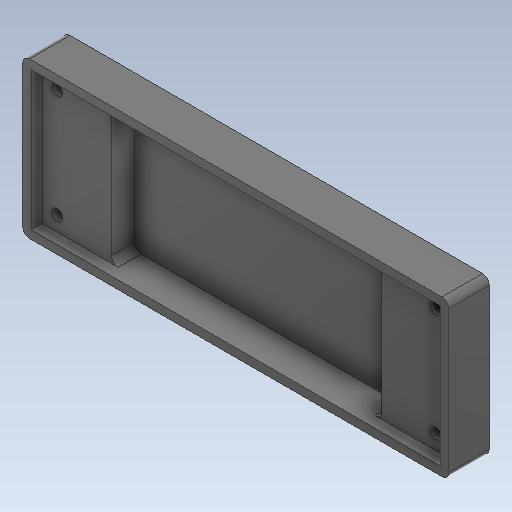
# Autodesk Inventor part: StartStopSwitch_cover_01
Saved by Autodesk Inventor 2020 (Build 240168000, 168)
## iProperties
Created: 2021-08-14
Part Number: StartStopSwitch_cover_01
Material: アセタール樹脂、黒
Document SubType Name: Modeling
Designer: Masato Kubotera
Density: 1.425 g/cm^3
Appearance: 滑らか - 黒
Mass: 5.48976 g
Surface Area: 46.7398 cm^2
Volume: 3.85246 cm^3
Author: Masato Kubotera
Title: StartStopSwitch_cover_01
Autodesk Inventor part; units mm, degrees
ref_plane "YZ Plane" through (0, 0, 0) normal (1, 0, 0) x (0, 1, 0)
ref_plane "XZ Plane" through (0, 0, 0) normal (0, 1, 0) x (-1, 0, 0)
ref_plane "XY Plane" through (0, 0, 0) normal (0, 0, 1) x (1, 0, 0)
sketch "スケッチ1" plane through (0, 0, 0) normal (0, 0, 1) x (1, 0, 0)
  line L0 (-31.5, 11.5) -> (31.5, 11.5)
  line L1 (31.5, 11.5) -> (31.5, -11.5)
  line L2 (31.5, -11.5) -> (-31.5, -11.5)
  line L3 (-31.5, -11.5) -> (-31.5, 11.5)
  line L4 (-31.5, 11.5) -> (31.5, -11.5) construction
  line L5 (31.5, 11.5) -> (-31.5, -11.5) construction
  line L6 (-30, 10) -> (30, 10) construction
  line L7 (30, 10) -> (30, -10) construction
  line L8 (30, -10) -> (-30, -10) construction
  line L9 (-30, -10) -> (-30, 10) construction
  line L10 (-30, 10) -> (30, -10) construction
  line L11 (30, 10) -> (-30, -10) construction
  circle A0 centre (-28, 8) radius 0.8
  line L12 (-31.5, 0) -> (31.5, 0) construction
  line L13 (0, 11.5) -> (0, -11.5) construction
  circle A1 centre (-28, -8) radius 0.8
  circle A2 centre (28, 8) radius 0.8
  circle A3 centre (28, -8) radius 0.8
  line L14 (-30.25, 10.25) -> (30.25, 10.25)
  line L15 (30.25, 10.25) -> (30.25, -10.25)
  line L16 (30.25, -10.25) -> (-30.25, -10.25)
  line L17 (-30.25, -10.25) -> (-30.25, 10.25)
  line L18 (-30.25, 10.25) -> (30.25, -10.25) construction
  line L19 (30.25, 10.25) -> (-30.25, -10.25) construction
  line L20 (-20, 10.25) -> (-20, -10.25)
  line L21 (20, 10.25) -> (20, -10.25)
  point P0 (0, 0)
  point P1 (0, 0)
  point P2 (20, -10.25)
  dimension "d0" = 63
  dimension "d1" = 60
  dimension "d2" = 20
  dimension "d3" = 23
  dimension "d4" = 1.6
  dimension "d5" = 2
  dimension "d6" = 2
  dimension "d7" = 20.5
  dimension "d8" = 60.5
  dimension "d13" = 10
  constraints: 44 end point, 12 midpoint, 6 parallel, 5 symmetric about line, 4 centre point, 4 perpendicular, 3 horizontal, 2 point on line, 3 other
  measures "d0" distance of L1.end L2.end
  measures "d1" distance of L7.end L8.end
  measures "d2" distance of L6.end L7.end
  measures "d3" distance of L0.end L1.end
  measures "d4" diameter of A0
  measures "d5" horizontal distance of A0.centre L6.start
  measures "d6" horizontal distance of A0.centre L6.start
  measures "d7" distance of L14.end L15.end
  measures "d8" distance of L15.end L16.end
  measures "d13" distance between parallel lines of L20 L9
extrude "押し出し1" add sketch "スケッチ1" against normal blind 1 contours L0 L1 L2 L3 | L14 L20 L16 L17 | L14 L21 L16 L20 | L14 L15 L16 L21
extrude "押し出し2" add sketch "スケッチ1" along normal blind 5 contours L0 L1 L2 L3
extrude "押し出し3" add sketch "スケッチ1" along normal blind 3.4 contours L14 L20 L16 L17 | L14 L15 L16 L21
fillet "フィレット1" radius 1 8 edges at (-31.5, -11.5, 2) (-31.5, 11.5, 2) (-20, 10.25, 1.7) (-20, -10.25, 1.7) (20, -10.25, 1.7) (20, 10.25, 1.7) (31.5, -11.5, 2) (31.5, 11.5, 2)
equation "\"d6\" = d5"
